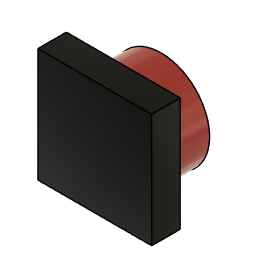
Boton (Autodesk Fusion 360 design; units mm, degrees)
Autodesk Fusion 360 part; units mm, degrees
sketch "Boceto1" plane through (0, 0, 0) normal (0, 1, 0) x (1, 0, 0)
  line L0 (6, 6) -> (-6, 6)
  line L1 (-6, 6) -> (-6, -6)
  line L2 (-6, -6) -> (6, -6)
  line L3 (6, -6) -> (6, 6)
  line L4 (6, 6) -> (-6, -6) construction
  line L5 (-6, 6) -> (6, -6) construction
  circle A0 centre (0, 0) radius 5.1025
  dimension "d2" = 12
  dimension "d3" = 12
  constraint horizontal L0
  constraint perpendicular L0 L1
  constraint parallel L0 L2
  constraint parallel L1 L3
  constraint coincident L4 A0.centre
  constraint coincident L5 A0.centre
  constraint coincident A0.centre origin
  measures "d2" distance of L1.end L2.end
  measures "d3" distance of L0.start L2.end
extrude "Extruir1" add sketch "Boceto1" along normal blind 4 contours A0
extrude "Extruir2" add sketch "Boceto1" against normal blind 3 contours L0 L1 L2 L3 | A0
